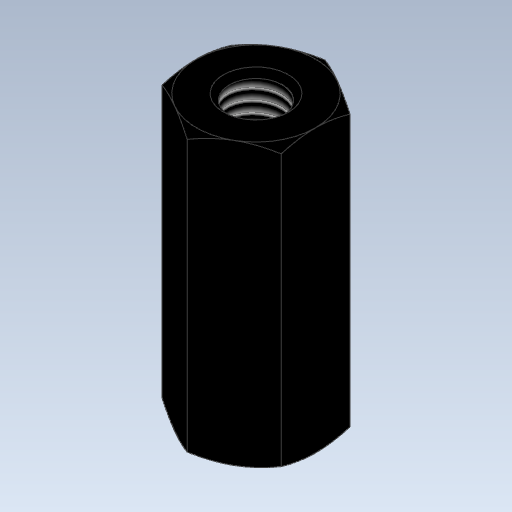
# Autodesk Inventor part: ASL-313BE
Saved by Autodesk Inventor 2020.4 (Build 244396000, 396)
## iProperties
Part Number: ASL-313BE
Material: アルミニウム 2014-T4
Document SubType Name: Modeling
Designer: Masato Kubotera
Density: 2.60204 g/cm^3
Appearance: 黒
Catalog Web Link: https://www.hirosugi-net.co.jp/shop/g/g13223/
Description: ReadyMade
Mass: 0.723 g
Surface Area: 3.86294 cm^2
Volume: 0.277859 cm^3
Author: Masato Kubotera
Autodesk Inventor part; units mm, degrees
ref_plane "YZ Plane" through (0, 0, 0) normal (1, 0, 0) x (0, 1, 0)
ref_plane "XZ Plane" through (0, 0, 0) normal (0, 1, 0) x (-1, 0, 0)
ref_plane "XY Plane" through (0, 0, 0) normal (0, 0, 1) x (1, 0, 0)
sketch "スケッチ1" plane through (0, 0, 0) normal (1, 0, 0) x (0, 1, 0)
  line L0 (-6.5, 0) -> (6.5, 0)
  line L1 (0, 0) -> (0, 3.1754) construction
  line L2 (-6.2544, 3.1754) -> (-6.5, 2.75)
  line L3 (-6.5, 2.75) -> (-6.5, 0)
  line L4 (-6.2544, 3.1754) -> (6.2544, 3.1754)
  line L5 (6.2544, 3.1754) -> (6.5, 2.75)
  line L6 (6.5, 2.75) -> (6.5, 0)
  dimension "d1" = 2.75
  dimension "d2" = 3.1754
  dimension "d3" = 30
  dimension "d4" = 13
  constraints: 14 end point, 3 perpendicular, 2 midpoint, 1 coincident, 1 horizontal, 1 symmetric about line
  measures "d1" distance of L0.start L2.end
  measures "d2" vertical distance of L0.start L2.start
  measures "d3" angle of L3 L2
  measures "d4" distance of L0.start L0.end
revolve "回転1" add sketch "スケッチ1" angle 360 about axis through (0, -6.5, 0) along (0, 1, 0)
sketch "スケッチ2" plane through (0, 6.5, 0) normal (0, 1, 0) x (1, 0, 0)
  circle A0 centre (0, 0) radius 3.1754 projected
  line L0 (0, -3.1754) -> (-2.75, -1.5877)
  line L1 (-2.75, -1.5877) -> (-2.75, 1.5877)
  line L2 (-2.75, 1.5877) -> (0, 3.1754)
  line L3 (0, 3.1754) -> (2.75, 1.5877)
  line L4 (2.75, 1.5877) -> (2.75, -1.5877)
  line L5 (2.75, -1.5877) -> (0, -3.1754)
  point P0 (0, 0)
  point P1 (0, 0)
  point P2 (2.75, -1.5877)
  point P3 (2.75, -1.5877)
  point P4 (2.75, 1.5877)
  point P5 (2.75, 1.5877)
  point P6 (0, 3.1754)
  point P7 (0, 3.1754)
  point P8 (-2.75, 1.5877)
  point P9 (-2.75, 1.5877)
  point P10 (-2.75, -1.5877)
  point P11 (-2.75, -1.5877)
  constraints: 12 end point, 2 coincident, 1 vertical, 15 other
extrude "押し出し1" cut sketch "スケッチ2" against normal through all contours A0 L4 | L3 A0 | A0 L5 | L2 A0 | A0 L0 | L1 A0
hole "穴1" at (0, 6.5, 0) direction (0, -1, 0) diameter 2.459 end through all countersink diameter 3 countersink angle 90 thread size "M3x0.5" class "6H" standard "ISO Metric profile"
mirror "ミラー1" about plane through (0, 0, 0) normal (0, 1, 0) of "穴1"
equation "\"d2\" = 1.1547 * d1"
